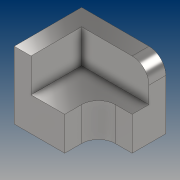
# Autodesk Inventor part: 36
Saved by Autodesk Inventor 2020.2 (Build 242310000, 310)
## iProperties
Created: 2020-09-17
Part Number: 36
Material: 鋼、碳鋼
Document SubType Name: Modeling
Designer: user
Density: 7.85 g/cm^3
Appearance: 半拋光
Mass: 378.485 g
Surface Area: 102.712 cm^2
Volume: 48.2146 cm^3
Author: user
Autodesk Inventor part; units mm, degrees
ref_plane "YZ Plane" through (0, 0, 0) normal (1, 0, 0) x (0, 1, 0)
ref_plane "XZ Plane" through (0, 0, 0) normal (0, 1, 0) x (-1, 0, 0)
ref_plane "XY Plane" through (0, 0, 0) normal (0, 0, 1) x (1, 0, 0)
sketch "草圖1" plane through (0, 0, 0) normal (0, 1, 0) x (-1, 0, 0)
  line L0 (0, 0) -> (-50, 0)
  line L1 (-50, 0) -> (-50, 40)
  line L2 (-50, 40) -> (0, 40)
  line L3 (0, 40) -> (0, 0)
  dimension "d0" = 50
  dimension "d2" = 40
  constraints: 8 end point, 2 parallel, 1 horizontal, 1 perpendicular
  measures "d0" distance of L1.end L2.end
  measures "d2" distance of L2.end L0.start
extrude "擠出1" add sketch "草圖1" along normal blind 40
sketch "草圖2" plane through (0, 0, 40) normal (0, 0, 1) x (1, 0, 0)
  line L0 (50, 40) -> (50, 0) projected
  line L1 (50, 0) -> (0, 0) projected
  line L2 (0, 0) -> (0, 40) projected
  line L3 (0, 40) -> (50, 40) projected
  line L4 (10, 59.2755) -> (53.3243, 59.2755)
  line L5 (53.3243, 59.2755) -> (53.3243, 20)
  line L6 (53.3243, 20) -> (10, 20)
  line L7 (10, 20) -> (10, 59.2755)
  dimension "d5" = 10
  dimension "d6" = 20
  constraints: 8 end point, 2 parallel, 1 horizontal, 1 perpendicular
  measures "d5" distance between parallel lines of L2 L7
  measures "d6" distance between parallel lines of L6 L3
extrude "擠出2" cut sketch "草圖2" against normal blind 30 contours L3 L7 L4 L5 L6 L0 | L0 L6 L7 L3
sketch "草圖3" plane through (10, 20, 40) normal (0, 1, 0) x (1, 0, 0)
  line L0 (40, 30) -> (0, 30) projected
  line L1 (0, 30) -> (0, 0) projected
  line L2 (40, 0) -> (0, 0) projected
  line L3 (40, 30) -> (40, 0) projected
  line L4 (40, 40) -> (40, 30) projected
  line L5 (-10, 40) -> (40, 40) projected
  line L6 (-10, 0) -> (-10, 40) projected
  line L7 (0, 0) -> (-10, 0) projected
  line L8 (-10, 0) -> (40, 0) projected
  line L9 (40, 0) -> (20, 0)
  line L10 (20, 0) -> (20, 20)
  line L11 (20, 20) -> (40, 20)
  line L12 (40, 20) -> (40, 0)
  point P0 (20, 0)
  dimension "d9" = 20
  dimension "d10" = 20
  constraints: 8 end point, 2 parallel, 1 horizontal, 1 perpendicular
  measures "d9" distance of L10.end L11.end
  measures "d10" distance of L9.end L10.end
extrude "擠出3" cut sketch "草圖3" against normal through all contours L3 L2 L10 L11
fillet "圓角1" radius 10 1 edges at (30, 10, 20)
fillet "圓角2" radius 10 1 edges at (50, 40, 5)
